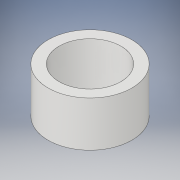
# Autodesk Inventor part: am-1306
Saved by Autodesk Inventor 2017.1 (Build 211199000, 199)
## iProperties
Category: Spacer
Company: Autodesk Inc.
Created: 2016-12-22
Part Number: am-1306
Material: Nylon 6/6
Document SubType Name: Modeling
Designer: Autodesk Inc.
Density: 1.13 g/cm^3
Appearance: Smooth - White
Catalog Web Link: http://www.andymark.com/product-p/am-1306.htm
Vendor: AndyMark Inc.
Author: Autodesk Inc.
Keywords: Drive Base Kit
Autodesk Inventor part; units mm, degrees
ref_plane "YZ Plane" through (0, 0, 0) normal (1, 0, 0) x (0, 1, 0)
ref_plane "XZ Plane" through (0, 0, 0) normal (0, 1, 0) x (-1, 0, 0)
ref_plane "XY Plane" through (0, 0, 0) normal (0, 0, 1) x (1, 0, 0)
sketch "Sketch1" plane through (0, 0, 0) normal (0, 1, 0) x (-1, 0, 0)
  circle A0 centre (0, 0) radius 6.5786
  dimension "d0" = 13.1572
  constraints: 1 centre point, 1 coincident
  measures "d0" diameter of A0
extrude "Extrusion1" add sketch "Sketch1" against normal blind 7.112
sketch "Sketch2" plane through (0, 0, 0) normal (0, 1, 0) x (1, 0, 0)
  circle A0 centre (0, 0) radius 4.8514
  dimension "d3" = 9.7028
  constraints: 1 centre point, 1 coincident
  measures "d3" diameter of A0
extrude "Extrusion2" cut sketch "Sketch2" against normal up to next
body "Solid1"
